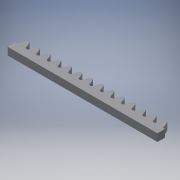
# Autodesk Inventor part: rack
Saved by Autodesk Inventor 2017 (Build 210142000, 142)
## iProperties
Created: 2018-01-02
Part Number: rack
Material: Generic
Document SubType Name: Modeling
Designer: RLanting
Density: 1 g/cm^3
Appearance: Default
Author: RLanting
Autodesk Inventor part; units mm, degrees
ref_plane "YZ Plane" through (0, 0, 0) normal (1, 0, 0) x (0, 1, 0)
ref_plane "XZ Plane" through (0, 0, 0) normal (0, 1, 0) x (-1, 0, 0)
ref_plane "XY Plane" through (0, 0, 0) normal (0, 0, 1) x (1, 0, 0)
sketch "Sketch1" plane through (0, 0, 0) normal (0, 0, 1) x (1, 0, 0)
  spline S0 degree 3 poles (-2.9605, 33.6199) (-2.8908, 33.5143) (-2.7514, 33.3031) (-2.5526, 32.9798) (-2.3616, 32.6518) (-2.1796, 32.3186) (-2.0074, 31.9804) (-1.8456, 31.637) (-1.6955, 31.2883) (-1.5581, 30.9344) (-1.4362, 30.575) (-1.3291, 30.2105) (-1.267, 29.9003) (-1.2143, 29.6528) (-1.1586, 29.4711) (-1.0848, 29.2961) (-0.9893, 29.1314) (-0.8888, 29.0086) (-0.7982, 28.9201) (-0.7221, 28.8633) (-0.6438, 28.8093) (-0.5576, 28.7691) (-0.4705, 28.7312) (-0.378, 28.709) (-0.2848, 28.6903) (-0.158, 28.6857) (0, 28.6887) (0.158, 28.6857) (0.2848, 28.6903) (0.378, 28.709) (0.4705, 28.7312) (0.5576, 28.7691) (0.6438, 28.8093) (0.7221, 28.8633) (0.7982, 28.9201) (0.8888, 29.0086) (0.9893, 29.1314) (1.0848, 29.2961) (1.1586, 29.4711) (1.2143, 29.6528) (1.267, 29.9003) (1.3291, 30.2105) (1.4362, 30.575) (1.5581, 30.9344) (1.6955, 31.2883) (1.8456, 31.637) (2.0074, 31.9804) (2.1796, 32.3186) (2.3616, 32.6518) (2.5526, 32.9798) (2.7514, 33.3031) (2.8908, 33.5143) (2.9605, 33.6199) knots 0 0 0 0 0.037953 0.075906 0.11386 0.151813 0.189766 0.227719 0.265671 0.303623 0.341574 0.379524 0.41747 0.436443 0.45541 0.474378 0.493341 0.512297 0.521786 0.531273 0.540758 0.550246 0.55973 0.569218 0.578704 0.58819 0.607167 0.626144 0.635631 0.645117 0.654605 0.664089 0.673577 0.683061 0.692549 0.702038 0.720994 0.739957 0.758925 0.777892 0.796865 0.834811 0.872761 0.910712 0.948664 0.986616 1.024569 1.062522 1.100475 1.138429 1.176382 1.214335 1.214335 1.214335 1.214335
  circle A0 centre (0, 0) radius 28.6875 construction
  circle A1 centre (0, 0) radius 29.6003 construction
  circle A2 centre (0, 0) radius 31.5 construction
  circle A3 centre (0, 0) radius 33.75
  line L0 (-2.9605, 33.6199) -> (2.9605, 33.6199)
  line L1 (2.9605, 33.6199) -> (2.9605, 38.6199)
  line L2 (2.9605, 38.6199) -> (-2.9605, 38.6199)
  line L3 (-2.9605, 38.6199) -> (-2.9605, 33.6199)
  point P0 (-2.7531, 33.302)
  point P1 (-2.5539, 32.979)
  point P2 (-2.3631, 32.6509)
  point P3 (-2.1812, 32.3178)
  point P4 (-2.0091, 31.9795)
  point P5 (-1.8475, 31.6361)
  point P6 (-1.6976, 31.2875)
  point P7 (-1.5607, 30.9335)
  point P8 (-1.4387, 30.5741)
  point P9 (-1.3345, 30.2092)
  point P10 (-1.2535, 29.8385)
  point P11 (-1.2116, 29.6535)
  point P12 (-1.1556, 29.4722)
  point P13 (-1.0812, 29.2978)
  point P14 (-0.9851, 29.1343)
  point P15 (-0.8654, 28.9873)
  point P16 (-0.7969, 28.9217)
  point P17 (-0.7217, 28.8637)
  point P18 (-0.6425, 28.8116)
  point P19 (-0.5575, 28.7695)
  point P20 (-0.4696, 28.7338)
  point P21 (-0.3779, 28.7096)
  point P22 (-0.2845, 28.6929)
  point P23 (-0.1898, 28.6875)
  point P24 (0, 28.6875)
  point P25 (0.1898, 28.6875)
  point P26 (0.2845, 28.6929)
  point P27 (0.3779, 28.7096)
  point P28 (0.4696, 28.7338)
  point P29 (0.5575, 28.7695)
  point P30 (0.6425, 28.8116)
  point P31 (0.7217, 28.8637)
  point P32 (0.7969, 28.9217)
  point P33 (0.8654, 28.9873)
  point P34 (0.9851, 29.1343)
  point P35 (1.0812, 29.2978)
  point P36 (1.1556, 29.4722)
  point P37 (1.2116, 29.6535)
  point P38 (1.2535, 29.8385)
  point P39 (1.3345, 30.2092)
  point P40 (1.4387, 30.5741)
  point P41 (1.5607, 30.9335)
  point P42 (1.6976, 31.2875)
  point P43 (1.8475, 31.6361)
  point P44 (2.0091, 31.9795)
  point P45 (2.1812, 32.3178)
  point P46 (2.3631, 32.6509)
  point P47 (2.5539, 32.979)
  point P48 (2.7531, 33.302)
  dimension "d6" = 5
  constraints: 8 end point, 4 centre point, 2 parallel, 2 point on circle, 1 horizontal, 1 perpendicular, 107 other
  measures "d6" distance of L0.end L1.end
sketch "Sketch2" plane through (0, 0, 0) normal (0, 0, 1) x (1, 0, 0)
  circle A0 centre (0, 0) radius 33.75 projected
  line L0 (-50, 33.6199) -> (50, 33.6199)
  line L1 (50, 33.6199) -> (50, 23.6199)
  line L2 (50, 23.6199) -> (-50, 23.6199)
  line L3 (-50, 23.6199) -> (-50, 33.6199)
  line L4 (-2.9605, 33.6199) -> (2.9605, 33.6199) projected
  point P0 (0, 33.6199)
  dimension "d2" = 100
  dimension "d3" = 10
  constraints: 8 end point, 2 midpoint, 2 parallel, 1 horizontal, 1 perpendicular
  measures "d2" distance of L1.end L2.end
  measures "d3" distance of L0.end L1.end
extrude "Extrusion2" add sketch "Sketch2" along normal blind 5 contours L0 L1 L2 A0 | A0 L2 L0 | A0 L2 L3 L0
extrude "Extrusion3" cut sketch "Sketch1" along normal through all contours L0 S0 | L3 L2 L1 A3 | A3 L0
pattern_linear "Rectangular Pattern1" count 15 spacing 7.065 along (-1, 0, 0) of "Extrusion3" first direction both ways yes
equation "\"Module\" = 2.25"
equation "\"PressureAngle\" = 20deg"
equation "\"UnitProfileClearance\" = 0.25"
equation "\"UnitRoundRadius\" = 0.35"
equation "\"HeadDiameter\" = 67.5"
equation "\"RootDiameter\" = 57.375"
equation "\"BaseDiameter\" = 59.20064"
equation "\"PitchDiameter\" = 63"
equation "\"HelixAngle\" = 0"
equation "\"UnitCorrection\" = 0"
equation "\"UnitAddendumModification\" = 0"
equation "\"CircularPitch\" = 7.068583"
equation "\"UnitBacklashShift\" = 0"
equation "\"TotalToolShift\" = 0"
equation "\"IsInternal\" = 0"
body "Solid2"
